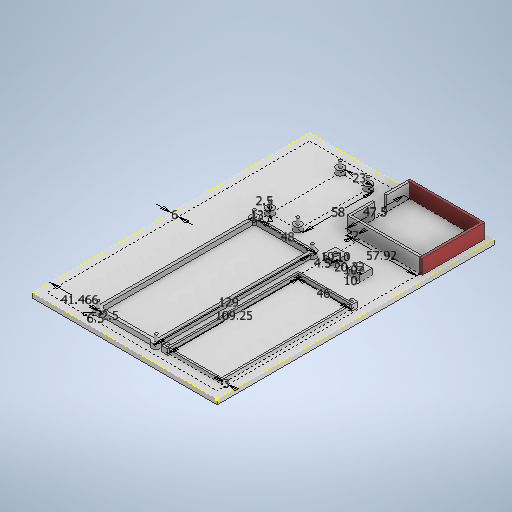
# Autodesk Inventor part: baseplate
Saved by Autodesk Inventor 2025 (Build 290162000, 162)
## iProperties
Created: 2025-05-12
Part Number: baseplate
Material: Generic
Document SubType Name: Modeling
Designer: ethan
Density: 1 g/cm^3
Appearance: Default
Author: ethan
Autodesk Inventor part; units mm, degrees
ref_plane "YZ Plane" through (0, 0, 0) normal (1, 0, 0) x (0, 1, 0)
ref_plane "XZ Plane" through (0, 0, 0) normal (0, 1, 0) x (-1, 0, 0)
ref_plane "XY Plane" through (0, 0, 0) normal (0, 0, 1) x (1, 0, 0)
sketch "Sketch1" plane through (0, 0, 0) normal (0, 1, 0) x (-1, 0, 0)
  line L0 (0, 0) -> (152.4, 0)
  line L1 (152.4, 0) -> (152.4, -228.6)
  line L2 (152.4, -228.6) -> (0, -228.6)
  line L3 (0, -228.6) -> (0, 0)
  dimension "d0" = 152.4
  dimension "d1" = 228.6
  constraints: 8 end point, 2 parallel, 1 horizontal, 1 perpendicular
  measures "d0" distance of L1.end L2.end
  measures "d1" distance of L0.end L1.end
extrude "Extrusion1" add sketch "Sketch1" along normal blind 4
sketch "Sketch2" plane through (0, 4, 0) normal (0, 1, 0) x (1, 0, 0)
  line L0 (0, 228.6) -> (-152.4, 228.6) construction
  line L1 (-152.4, 228.6) -> (-152.4, 0) construction
  line L2 (-152.4, 0) -> (0, 0) construction
  line L3 (0, 0) -> (0, 228.6) construction
  line L4 (-146.4, 6) -> (-146.4, 222.6) construction
  line L5 (-146.4, 222.6) -> (-6, 222.6) construction
  line L6 (-6, 222.6) -> (-6, 6) construction
  line L7 (-6, 6) -> (-146.4, 6) construction
  line L8 (-110.934, 6) -> (-110.934, 12.5) construction
  circle A0 centre (-110.934, 12.5) radius 1.25 construction
  line L9 (-110.934, 12.5) -> (-62.934, 12.5) construction
  line L10 (-62.934, 12.5) -> (-62.934, 141.5) construction
  line L11 (-62.934, 141.5) -> (-110.934, 141.5) construction
  line L12 (-110.934, 141.5) -> (-110.934, 12.5) construction
  circle A1 centre (-62.934, 12.5) radius 1.25 construction
  circle A2 centre (-110.934, 141.5) radius 1.25 construction
  circle A3 centre (-62.934, 141.5) radius 1.25 construction
  line L13 (-62.934, 12.5) -> (-6, 12.5) construction
  line L14 (-6, 12.5) -> (-9, 12.5) construction
  line L15 (-9, 12.5) -> (-55, 12.5) construction
  line L16 (-55, 12.5) -> (-55, 121.75) construction
  line L17 (-55, 121.75) -> (-9, 121.75) construction
  line L18 (-9, 121.75) -> (-9, 12.5) construction
  line L19 (-6, 222.6) -> (-63.92, 222.6) construction
  line L20 (-63.92, 222.6) -> (-63.92, 175.1) construction
  line L21 (-63.92, 175.1) -> (-6, 175.1) construction
  line L22 (-6, 175.1) -> (-6, 222.6) construction
  line L23 (-63.92, 222.6) -> (-65.92, 222.6) construction
  line L24 (-65.92, 222.6) -> (-65.92, 175.1) construction
  line L25 (-65.92, 175.1) -> (-63.92, 175.1) construction
  line L26 (-63.92, 175.1) -> (-63.92, 222.6) construction
  line L27 (-63.92, 175.1) -> (-6, 175.1) construction
  line L28 (-6, 175.1) -> (-6, 173.1) construction
  line L29 (-6, 173.1) -> (-63.92, 173.1) construction
  line L30 (-63.92, 173.1) -> (-63.92, 175.1) construction
  line L31 (-63.92, 175.1) -> (-65.92, 175.1) construction
  line L32 (-65.92, 175.1) -> (-65.92, 173.1) construction
  line L33 (-65.92, 173.1) -> (-63.92, 173.1) construction
  line L34 (-63.92, 173.1) -> (-63.92, 175.1) construction
  line L35 (-55, 121.75) -> (-55, 173.1) construction
  line L36 (-110.934, 141.5) -> (-110.934, 154.5) construction
  circle A4 centre (-110.934, 154.5) radius 1.25 construction
  line L37 (-110.934, 154.5) -> (-87.934, 154.5) construction
  line L38 (-87.934, 154.5) -> (-87.934, 212.5) construction
  line L39 (-87.934, 212.5) -> (-110.934, 212.5) construction
  line L40 (-110.934, 212.5) -> (-110.934, 154.5) construction
  circle A5 centre (-87.934, 154.5) radius 1.25 construction
  circle A6 centre (-87.934, 212.5) radius 1.25 construction
  circle A7 centre (-110.934, 212.5) radius 1.25 construction
  line L41 (-45, 142.425) -> (-55, 142.425) construction
  line L42 (-55, 142.425) -> (-55, 152.425) construction
  line L43 (-55, 152.425) -> (-45, 152.425) construction
  line L44 (-45, 152.425) -> (-45, 142.425) construction
  line L45 (-45, 142.425) -> (-55, 152.425) construction
  line L46 (-55, 142.425) -> (-45, 152.425) construction
  circle A8 centre (-50, 147.425) radius 2.25 construction
  line L47 (-50, 147.425) -> (-29.68, 147.425) construction
  line L48 (-24.68, 152.425) -> (-34.68, 152.425) construction
  line L49 (-34.68, 152.425) -> (-34.68, 142.425) construction
  line L50 (-34.68, 142.425) -> (-24.68, 142.425) construction
  line L51 (-24.68, 142.425) -> (-24.68, 152.425) construction
  line L52 (-24.68, 152.425) -> (-34.68, 142.425) construction
  line L53 (-34.68, 152.425) -> (-24.68, 142.425) construction
  dimension "d4" = 6
  dimension "d6" = 6.5
  dimension "d7" = 2.5
  dimension "d8" = 48
  dimension "d9" = 129
  dimension "d14" = 3
  dimension "d15" = 46
  dimension "d16" = 109.25
  dimension "d17" = 41.466
  dimension "d18" = 57.92
  dimension "d19" = 47.5
  dimension "d29" = 13
  dimension "d30" = 2.5
  dimension "d31" = 23
  dimension "d32" = 58
  dimension "d33" = 2
  dimension "d64" = 10
  dimension "d65" = 10
  dimension "d66" = 4.5
  dimension "d67" = 20.32
  dimension "d68" = 10
  dimension "d69" = 10
  constraints: 100 end point, 18 parallel, 12 perpendicular, 10 horizontal, 9 centre point, 8 coincident, 8 point on line, 2 midpoint, 3 other
  measures "d4" distance between parallel lines of L1 L4
  measures "d6" distance of L8.start L8.end
  measures "d7" diameter of A0
  measures "d8" distance of L11.end L10.end
  measures "d9" distance of L10.end L9.end
  measures "d14" distance of L13.end L14.end
  measures "d15" distance of L16.end L17.end
  measures "d16" distance of L15.end L16.end
  measures "d17" distance between parallel lines of L1 L12
  measures "d18" distance of L21.end L20.end
  measures "d19" distance of L20.end L19.end
  measures "d29" distance of L36.start L36.end
  measures "d30" diameter of A4
  measures "d31" distance of L39.end L38.end
  measures "d32" distance of L38.end L37.end
  measures "d33" distance between parallel lines of L29 L21
  measures "d64" distance of L42.end L43.end
  measures "d65" distance of L41.end L42.end
  measures "d66" diameter of A8
  measures "d67" distance of L47.start L47.end
  measures "d68" distance of L50.end L49.end
  measures "d69" distance of L49.end L48.end
sketch "Sketch3" plane through (0, 4, 0) normal (0, 1, 0) x (1, 0, 0)
  circle A0 centre (-110.934, 12.5) radius 1.25 construction
  circle A1 centre (-110.934, 141.5) radius 1.25 construction
  circle A2 centre (-62.934, 141.5) radius 1.25 construction
  circle A3 centre (-62.934, 12.5) radius 1.25 construction
  circle A4 centre (-110.934, 12.5) radius 3.25
  circle A5 centre (-110.934, 141.5) radius 3.25
  circle A6 centre (-62.934, 141.5) radius 3.25
  circle A7 centre (-62.934, 12.5) radius 3.25
  point P0 (0, 0)
  dimension "d37" = 2
  dimension "d38" = 2
  dimension "d39" = 2
  dimension "d40" = 2
  constraints: 4 centre point
  measures "d37" radial gap between concentric circles of A0 A4
  measures "d38" radial gap between concentric circles of A1 A5
  measures "d39" radial gap between concentric circles of A2 A6
  measures "d40" radial gap between concentric circles of A3 A7
extrude "Extrusion2" add sketch "Sketch3" along normal blind 4
sketch "Sketch4" plane through (-110.934, 8, -12.5) normal (0, 1, 0) x (1, 0, 0)
  circle A0 centre (0, 0) radius 3.25 projected
  circle A1 centre (0, 129) radius 3.25 projected
  circle A2 centre (48, 129) radius 3.25 projected
  circle A3 centre (48, 0) radius 3.25 projected
  circle A4 centre (48, 0) radius 1.25
  circle A5 centre (0, 0) radius 1.25
  circle A6 centre (0, 129) radius 1.25
  circle A7 centre (48, 129) radius 1.25
  point P0 (110.934, -12.5)
  dimension "d43" = 2.5
  dimension "d44" = 2.5
  dimension "d45" = 2.5
  dimension "d46" = 2.5
  constraints: 4 centre point, 4 coincident
  measures "d43" diameter of A4
  measures "d44" diameter of A5
  measures "d45" diameter of A6
  measures "d46" diameter of A7
extrude "Extrusion3" add sketch "Sketch4" along normal blind 5 contours A4 | A5 | A6 | A7
sketch "Sketch5" plane through (0, 4, 0) normal (0, 1, 0) x (1, 0, 0)
  circle A0 centre (-110.934, 154.5) radius 1.25 construction
  circle A1 centre (-110.934, 212.5) radius 1.25 construction
  circle A2 centre (-87.934, 212.5) radius 1.25 construction
  line L0 (-87.934, 154.5) -> (-87.934, 212.5) construction
  circle A3 centre (-87.934, 154.5) radius 1.25 construction
  circle A4 centre (-87.934, 154.5) radius 3.25
  circle A5 centre (-110.934, 154.5) radius 3.25
  circle A6 centre (-110.934, 212.5) radius 3.25
  circle A7 centre (-87.934, 212.5) radius 3.25
  point P0 (0, 0)
  dimension "d49" = 2
  dimension "d50" = 2
  dimension "d51" = 2
  dimension "d52" = 2
  constraints: 4 centre point
  measures "d49" radial gap between concentric circles of A3 A4
  measures "d50" radial gap between concentric circles of A0 A5
  measures "d51" radial gap between concentric circles of A1 A6
  measures "d52" radial gap between concentric circles of A2 A7
extrude "Extrusion4" add sketch "Sketch5" along normal blind 4
sketch "Sketch6" plane through (-87.934, 8, -154.5) normal (0, 1, 0) x (1, 0, 0)
  circle A0 centre (-23, 0) radius 3.25 construction
  circle A1 centre (-23, 58) radius 3.25 construction
  circle A2 centre (0, 58) radius 3.25 construction
  circle A3 centre (0, 0) radius 3.25 construction
  circle A4 centre (-23, 0) radius 1.25
  circle A5 centre (-23, 58) radius 1.25
  circle A6 centre (0, 58) radius 1.25
  circle A7 centre (0, 0) radius 1.25
  point P0 (87.934, -154.5)
  dimension "d55" = 2.5
  dimension "d56" = 2.5
  dimension "d57" = 2.5
  dimension "d58" = 2.5
  constraints: 4 centre point, 4 coincident
  measures "d55" diameter of A4
  measures "d56" diameter of A5
  measures "d57" diameter of A6
  measures "d58" diameter of A7
extrude "Extrusion5" add sketch "Sketch6" along normal blind 5
sketch "Sketch7" plane through (0, 4, 0) normal (0, 1, 0) x (1, 0, 0)
  line L0 (-45, 142.425) -> (-55, 142.425) construction
  line L1 (-45, 152.425) -> (-45, 142.425) construction
  line L2 (-34.68, 152.425) -> (-34.68, 142.425) construction
  line L3 (-34.68, 142.425) -> (-24.68, 142.425) construction
  line L4 (-45, 142.425) -> (-55, 142.425)
  line L5 (-55, 142.425) -> (-55, 152.425)
  line L6 (-55, 152.425) -> (-45, 152.425)
  line L7 (-45, 152.425) -> (-45, 142.425)
  line L8 (-34.68, 142.425) -> (-24.68, 142.425)
  line L9 (-24.68, 142.425) -> (-24.68, 152.425)
  line L10 (-24.68, 152.425) -> (-34.68, 152.425)
  line L11 (-34.68, 152.425) -> (-34.68, 142.425)
  point P0 (0, 0)
  constraints: 16 end point, 4 parallel, 2 horizontal, 2 perpendicular, 1 point on line
extrude "Extrusion6" add sketch "Sketch7" along normal blind 5
sketch "Sketch8" plane through (0, 9, 0) normal (0, 1, 0) x (1, 0, 0)
  line L0 (-45, 152.425) -> (-55, 152.425) projected
  line L1 (-55, 152.425) -> (-55, 142.425) projected
  line L2 (-55, 142.425) -> (-45, 142.425) projected
  line L3 (-45, 142.425) -> (-45, 152.425) projected
  line L4 (-24.68, 142.425) -> (-24.68, 152.425) projected
  line L5 (-24.68, 152.425) -> (-34.68, 152.425) projected
  line L6 (-34.68, 152.425) -> (-34.68, 142.425) projected
  line L7 (-34.68, 142.425) -> (-24.68, 142.425) projected
  circle A0 centre (-50, 147.425) radius 2.25
  circle A1 centre (-29.68, 147.425) radius 2.25
  point P0 (0, 0)
  dimension "d72" = 4.5
  dimension "d73" = 4.5
  constraints: 2 centre point
  measures "d72" diameter of A0
  measures "d73" diameter of A1
extrude "Extrusion7" cut sketch "Sketch8" against normal blind 5 contours A0 | A1
sketch "Sketch9" plane through (0, 4, 0) normal (0, 1, 0) x (1, 0, 0)
  line L0 (-55, 12.5) -> (-55, 121.75) construction
  line L1 (-9, 12.5) -> (-55, 12.5) construction
  line L2 (-55, 12.5) -> (-9, 12.5)
  line L3 (-9, 12.5) -> (-9, 121.75)
  line L4 (-9, 121.75) -> (-55, 121.75)
  line L5 (-55, 121.75) -> (-55, 12.5)
  line L6 (-53.4, 121.75) -> (-53.4, 14.1)
  line L7 (-53.4, 14.1) -> (-9, 14.1)
  line L8 (-53.4, 120.15) -> (-10.6, 120.15)
  line L9 (-10.6, 120.15) -> (-10.6, 14.1)
  line L10 (-10.6, 14.1) -> (-53.4, 14.1)
  line L11 (-53.4, 14.1) -> (-53.4, 120.15)
  point P0 (0, 0)
  dimension "d76" = 1.6
  dimension "d77" = 1.6
  constraints: 20 end point, 4 parallel, 2 perpendicular, 1 horizontal, 4 other
  measures "d76" distance between parallel lines of L0 L6
  measures "d77" distance between parallel lines of L4 L8
extrude "Extrusion8" add sketch "Sketch9" along normal blind 3 contours L5 L4 L6 L7 L3 L2 | L7 L9 L8 L6 L4 L3
sketch "Sketch10" plane through (0, 4, 0) normal (0, 1, 0) x (1, 0, 0)
  line L0 (-55, 121.75) -> (-55, 12.5) construction
  line L1 (-55, 12.5) -> (-9, 12.5) construction
  line L2 (-9, 12.5) -> (-9, 121.75) construction
  line L3 (-9, 121.75) -> (-55, 121.75) construction
  line L4 (-53.4, 120.15) -> (-10.6, 120.15) construction
  line L5 (-10.6, 120.15) -> (-10.6, 14.1) construction
  line L6 (-10.6, 14.1) -> (-53.4, 14.1) construction
  line L7 (-53.4, 14.1) -> (-53.4, 120.15) construction
  line L8 (-56.6, 10.9) -> (-56.6, 123.35) construction
  line L9 (-56.6, 123.35) -> (-7.4, 123.35) construction
  line L10 (-7.4, 123.35) -> (-7.4, 10.9) construction
  line L11 (-7.4, 10.9) -> (-56.6, 10.9) construction
  line L12 (-56.6, 10.9) -> (-51.6, 10.9) construction
  line L13 (-51.6, 10.9) -> (-51.6, 15.9) construction
  line L14 (-51.6, 15.9) -> (-56.6, 15.9) construction
  line L15 (-56.6, 15.9) -> (-56.6, 10.9) construction
  line L16 (-51.6, 10.9) -> (-51.6, 12.5)
  line L17 (-55, 12.5) -> (-51.6, 12.5)
  line L18 (-55, 12.5) -> (-55, 15.9)
  line L19 (-55, 15.9) -> (-56.6, 15.9)
  line L20 (-56.6, 15.9) -> (-56.6, 10.9)
  line L21 (-56.6, 10.9) -> (-51.6, 10.9)
  line L22 (-7.4, 123.35) -> (-12.4, 123.35)
  line L23 (-12.4, 123.35) -> (-12.4, 118.35)
  line L24 (-12.4, 118.35) -> (-7.4, 118.35)
  line L25 (-7.4, 118.35) -> (-7.4, 123.35)
  line L26 (-9, 121.75) -> (-55, 121.75) projected
  line L27 (-12.4, 121.75) -> (-9, 121.75)
  line L28 (-9, 121.75) -> (-9, 118.35)
  point P0 (0, 0)
  dimension "d80" = 1.6
  dimension "d81" = 5
  dimension "d82" = 5
  dimension "d83" = 5
  dimension "d84" = 5
  constraints: 40 end point, 8 point on line, 4 parallel, 4 perpendicular, 3 collinear, 2 horizontal, 3 other
  measures "d80" distance between parallel lines of L0 L8
  measures "d81" distance of L14.end L13.end
  measures "d82" distance of L13.end L12.end
  measures "d83" distance of L24.end L23.end
  measures "d84" distance of L23.end L22.end
extrude "Extrusion9" add sketch "Sketch10" along normal blind 4.5 contours L21 L20 L19 L18 L17 L16 | L25 L24 L28 L26 L23 L22
sketch "Sketch11" plane through (0, 4, 0) normal (0, 1, 0) x (1, 0, 0)
  line L0 (-65.92, 222.6) -> (-65.92, 175.1) construction
  line L1 (-63.92, 222.6) -> (-63.92, 175.1) construction
  line L2 (-63.92, 175.1) -> (-6, 175.1) construction
  line L3 (-6, 173.1) -> (-63.92, 173.1) construction
  line L4 (-65.92, 173.1) -> (-63.92, 173.1) construction
  line L5 (-65.92, 175.1) -> (-65.92, 173.1) construction
  line L6 (-65.92, 173.1) -> (-6, 173.1)
  line L7 (-6, 173.1) -> (-6, 222.6)
  line L8 (-6, 222.6) -> (-65.92, 222.6)
  line L9 (-65.92, 222.6) -> (-65.92, 173.1)
  line L10 (-63.92, 175.1) -> (-6, 175.1)
  line L11 (-6, 175.1) -> (-6, 222.6)
  line L12 (-6, 222.6) -> (-63.92, 222.6)
  line L13 (-63.92, 222.6) -> (-63.92, 175.1)
  point P0 (0, 0)
  constraints: 16 end point, 4 parallel, 2 horizontal, 2 perpendicular
extrude "Extrusion10" add sketch "Sketch11" along normal blind 12 contours L9 L8 L13 L10 L7 L6
sketch "Sketch12" plane through (0, 16, 0) normal (0, 1, 0) x (1, 0, 0)
  line L0 (-63.92, 175.1) -> (-63.92, 222.6) projected
  line L1 (-59.9316, 193.85) -> (-59.9316, 203.85)
  line L2 (-59.9316, 203.85) -> (-67.9084, 203.85)
  line L3 (-67.9084, 203.85) -> (-67.9084, 193.85)
  line L4 (-67.9084, 193.85) -> (-59.9316, 193.85)
  line L5 (-59.9316, 193.85) -> (-67.9084, 203.85) construction
  line L6 (-59.9316, 203.85) -> (-67.9084, 193.85) construction
  point P0 (0, 0)
  point P1 (-63.92, 198.85)
  point P2 (-63.92, 193.85)
  point P3 (-63.92, 203.85)
  dimension "d89" = 10
  constraints: 12 end point, 3 midpoint, 2 parallel, 1 perpendicular
  measures "d89" distance of L1.start L1.end
extrude "Extrusion11" cut sketch "Sketch12" against normal blind 12 contours L4 L3 L2 L0
sketch "Sketch13" plane through (0, 4, 0) normal (0, 1, 0) x (1, 0, 0)
  line L0 (-63.92, 193.85) -> (-63.92, 175.1) projected
  line L1 (-63.92, 175.1) -> (-6, 175.1) projected
  line L2 (-6, 175.1) -> (-6, 173.1) projected
  line L3 (-6, 173.1) -> (-65.92, 173.1) projected
  line L4 (-65.92, 173.1) -> (-65.92, 193.85) projected
  line L5 (-63.92, 193.85) -> (-65.92, 193.85) projected
  line L6 (-65.92, 203.85) -> (-63.92, 203.85) projected
  line L7 (-65.92, 203.85) -> (-65.92, 222.6) projected
  line L8 (-65.92, 222.6) -> (-63.92, 222.6) projected
  line L9 (-63.92, 222.6) -> (-63.92, 203.85) projected
  line L10 (-51.6, 12.5) -> (-51.6, 10.9) projected
  line L11 (-51.6, 10.9) -> (-56.6, 10.9) projected
  line L12 (-56.6, 10.9) -> (-56.6, 15.9) projected
  line L13 (-56.6, 15.9) -> (-55, 15.9) projected
  line L14 (-55, 15.9) -> (-55, 121.75) projected
  line L15 (-55, 121.75) -> (-12.4, 121.75) projected
  line L16 (-12.4, 121.75) -> (-12.4, 123.35) projected
  line L17 (-12.4, 123.35) -> (-7.4, 123.35) projected
  line L18 (-7.4, 123.35) -> (-7.4, 118.35) projected
  line L19 (-7.4, 118.35) -> (-9, 118.35) projected
  line L20 (-9, 118.35) -> (-9, 12.5) projected
  line L21 (-9, 12.5) -> (-51.6, 12.5) projected
  line L22 (-24.68, 142.425) -> (-34.68, 142.425) projected
  line L23 (-34.68, 142.425) -> (-34.68, 152.425) projected
  line L24 (-34.68, 152.425) -> (-24.68, 152.425) projected
  line L25 (-24.68, 152.425) -> (-24.68, 142.425) projected
  line L26 (-45, 152.425) -> (-45, 142.425) projected
  line L27 (-45, 142.425) -> (-55, 142.425) projected
  line L28 (-55, 142.425) -> (-55, 152.425) projected
  line L29 (-55, 152.425) -> (-45, 152.425) projected
  circle A0 centre (-110.934, 212.5) radius 3.25 projected
  circle A1 centre (-110.934, 154.5) radius 3.25 projected
  circle A2 centre (-87.934, 154.5) radius 3.25 projected
  circle A3 centre (-87.934, 212.5) radius 3.25 projected
  circle A4 centre (-62.934, 141.5) radius 3.25 projected
  circle A5 centre (-110.934, 141.5) radius 3.25 projected
  circle A6 centre (-110.934, 12.5) radius 3.25 projected
  circle A7 centre (-62.934, 12.5) radius 3.25 projected
  line L30 (0, 228.6) -> (-152.4, 228.6) projected
  line L31 (-152.4, 228.6) -> (-152.4, 0) projected
  line L32 (-152.4, 0) -> (0, 0) projected
  line L33 (0, 0) -> (0, 228.6) projected
  line L34 (-65.92, 222.6) -> (-6, 222.6)
  line L35 (-6, 222.6) -> (-6, 224.6)
  line L36 (-6, 224.6) -> (-65.92, 224.6)
  line L37 (-65.92, 224.6) -> (-65.92, 222.6)
  line L38 (-6, 224.6) -> (-4, 224.6)
  line L39 (-4, 224.6) -> (-4, 173.1)
  line L40 (-4, 173.1) -> (-6, 173.1)
  line L41 (-6, 173.1) -> (-6, 224.6)
  dimension "d92" = 2
  dimension "d93" = 2
  constraints: 16 end point, 4 parallel, 2 horizontal, 2 perpendicular
  measures "d92" distance of L35.end L34.end
  measures "d93" distance of L39.end L40.end
extrude "Extrusion12" add sketch "Sketch13" along normal blind 12 separate body contours L41 L35 L38 L39 L40 L2 | L34 L8 L37 L36 L35
sketch "Sketch14" plane through (0, 4, 0) normal (0, 1, 0) x (1, 0, 0)
  circle A0 centre (-62.934, 141.5) radius 1.25 projected
  circle A1 centre (-62.934, 12.5) radius 1.25 projected
  circle A2 centre (-110.934, 12.5) radius 1.25 projected
  circle A3 centre (-110.934, 141.5) radius 1.25 projected
  line L0 (-62.934, 142.75) -> (-110.934, 142.75)
  circle A4 centre (-62.934, 141.5) radius 1.25 projected
  line L1 (-112.184, 141.5) -> (-112.184, 12.5)
  line L2 (-110.934, 11.25) -> (-62.934, 11.25)
  line L3 (-61.684, 12.5) -> (-61.684, 141.5)
  line L4 (-61.684, 142.75) -> (-64.184, 142.75) construction
  line L5 (-64.184, 142.75) -> (-64.184, 140.25) construction
  line L6 (-64.184, 140.25) -> (-61.684, 140.25) construction
  line L7 (-61.684, 140.25) -> (-61.684, 142.75) construction
  line L8 (-64.184, 140.25) -> (-110.934, 140.25) construction
  line L9 (-64.184, 141.5) -> (-64.184, 12.5)
  line L10 (-62.934, 13.75) -> (-110.934, 13.75)
  line L11 (-109.684, 12.5) -> (-109.684, 141.5)
  line L12 (-110.934, 140.25) -> (-62.934, 140.25)
  point P0 (0, 0)
  point P1 (-64.184, 13.75)
  point P2 (-109.684, 140.25)
  point P3 (-109.684, 13.75)
  constraints: 26 end point, 13 point on circle, 8 tangent, 4 horizontal, 2 midpoint, 2 parallel, 1 perpendicular, 1 point on line, 2 other
extrude "Extrusion13" add sketch "Sketch14" along normal blind 4 contours L3 A1 L10 L9 L12 A0 | A0 L9 L12 L11 A3 L0 | L2 A2 L11 L10 L9 A1 | A3 L12 L11 L10 A2 L1 bodies 1
body "Solid1"
body "Solid2"
